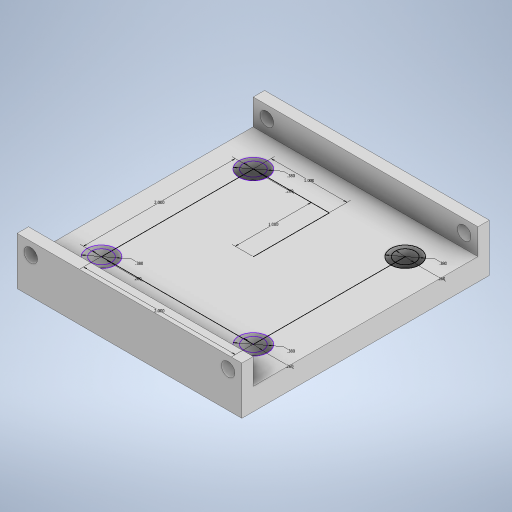
# Autodesk Inventor part: Voicecoil_to_PY004_Coupler
Saved by Autodesk Inventor 2024.2 (Build 282272000, 272)
## iProperties
Created: 2023-11-10
Part Number: Voicecoil_to_PY004_Coupler
Material: Generic
Document SubType Name: Modeling
Designer: S227943
Density: 1 g/cm^3
Appearance: Default
Author: S227943
Autodesk Inventor part; units mm, degrees
ref_plane "YZ Plane" through (0, 0, 0) normal (1, 0, 0) x (0, 1, 0)
ref_plane "XZ Plane" through (0, 0, 0) normal (0, 1, 0) x (-1, 0, 0)
ref_plane "XY Plane" through (0, 0, 0) normal (0, 0, 1) x (1, 0, 0)
sketch "Sketch1" plane through (0, 0, 0) normal (0, 1, 0) x (-1, 0, 0)
  line L0 (37.592, 37.592) -> (-37.592, 37.592)
  line L1 (-37.592, 37.592) -> (-37.592, -37.592)
  line L2 (-37.592, -37.592) -> (37.592, -37.592)
  line L3 (37.592, -37.592) -> (37.592, 37.592)
  line L4 (48.9249, 50.7063) -> (48.9249, -4.5387)
  line L5 (37.592, 0) -> (0, 0)
  line L6 (0, 0) -> (0, -37.592)
  point P0 (0, 0)
  dimension "d0" = 75.184
  dimension "d1" = 75.184
  constraints: 14 end point, 3 parallel, 2 midpoint, 1 horizontal, 1 perpendicular
  measures "d0" distance of L1.end L2.end
  measures "d1" distance of L0.end L1.end
extrude "Extrusion1" add sketch "Sketch1" along normal blind 7.366
sketch "Sketch6" plane through (0, 7.366, 0) normal (0, 1, 0) x (1, 0, 0)
  line L0 (0, 0) -> (0, 25.4)
  line L1 (0, 25.4) -> (-25.4, 25.4)
  line L2 (-25.4, 25.4) -> (-25.4, -25.4)
  line L3 (-25.4, -25.4) -> (25.4, -25.4)
  line L4 (25.4, -25.4) -> (25.4, 25.4)
  circle A0 centre (25.4, 25.4) radius 3.302
  circle A1 centre (25.4, 25.4) radius 4.826
  circle A2 centre (25.4, -25.4) radius 3.302
  circle A3 centre (25.4, -25.4) radius 4.826
  circle A4 centre (-25.4, -25.4) radius 3.302
  circle A5 centre (-25.4, -25.4) radius 4.826
  circle A6 centre (-25.4, 25.4) radius 3.302
  circle A7 centre (-25.4, 25.4) radius 4.826
  dimension "d35" = 25.4
  dimension "d36" = 25.4
  dimension "d37" = 50.8
  dimension "d38" = 50.8
  dimension "d39" = 6.604
  dimension "d40" = 9.652
  dimension "d41" = 6.604
  dimension "d42" = 9.652
  dimension "d43" = 6.604
  dimension "d44" = 9.652
  dimension "d45" = 6.604
  dimension "d46" = 9.652
  constraints: 10 end point, 8 centre point, 8 coincident, 4 perpendicular, 1 point on line, 1 vertical
  measures "d35" distance of L0.start L0.end
  measures "d36" distance of L0.end L1.end
  measures "d37" distance of L1.end L2.end
  measures "d38" distance of L2.end L3.end
  measures "d39" diameter of A0
  measures "d40" diameter of A1
  measures "d41" diameter of A2
  measures "d42" diameter of A3
  measures "d43" diameter of A4
  measures "d44" diameter of A5
  measures "d45" diameter of A6
  measures "d46" diameter of A7
sketch "Sketch2" plane through (0, 7.366, 0) normal (0, 1, 0) x (1, 0, 0)
  line L0 (0, 0) -> (0, 12.7)
  line L1 (0, 12.7) -> (-12.7, 12.7)
  line L2 (-12.7, 12.7) -> (12.7, 12.7)
  line L3 (12.7, 12.7) -> (12.7, -12.7)
  line L4 (12.7, -12.7) -> (-12.7, -12.7)
  circle A0 centre (-12.7, -12.7) radius 3.302
  circle A1 centre (-12.7, -12.7) radius 4.826
  circle A2 centre (-12.7, 12.7) radius 3.302
  circle A3 centre (-12.7, 12.7) radius 4.826
  circle A4 centre (12.7, -12.7) radius 3.302
  circle A5 centre (12.7, -12.7) radius 4.826
  circle A6 centre (12.7, 12.7) radius 3.302
  circle A7 centre (12.7, 12.7) radius 4.826
  dimension "d4" = 12.7
  dimension "d5" = 12.7
  dimension "d6" = 25.4
  dimension "d7" = 25.4
  dimension "d8" = 25.4
  dimension "d9" = 6.604
  dimension "d10" = 9.652
  dimension "d11" = 6.604
  dimension "d12" = 9.652
  dimension "d13" = 6.604
  dimension "d14" = 9.652
  dimension "d15" = 6.604
  dimension "d16" = 9.652
  constraints: 10 end point, 8 centre point, 5 coincident, 3 perpendicular, 1 point on line, 1 vertical
  measures "d4" distance of L0.start L0.end
  measures "d5" distance of L0.end L1.end
  measures "d6" distance of L1.end L2.end
  measures "d7" distance of L2.end L3.end
  measures "d8" distance of L3.end L4.end
  measures "d9" diameter of A0
  measures "d10" diameter of A1
  measures "d11" diameter of A2
  measures "d12" diameter of A3
  measures "d13" diameter of A4
  measures "d14" diameter of A5
  measures "d15" diameter of A6
  measures "d16" diameter of A7
sketch "Sketch3" plane through (-37.592, 0, 37.592) normal (0, 0, 1) x (1, 0, 0)
  point P0 (37.592, 0)
sketch "Sketch4" plane through (0, 0, 0) normal (0, -1, 0) x (1, 0, 0)
  line L0 (-37.592, 37.592) -> (38.608, 37.592)
  line L1 (38.608, 37.592) -> (38.608, 41.402)
  line L2 (38.608, 41.402) -> (-37.592, 41.402)
  line L3 (-37.592, 41.402) -> (-37.592, 37.592)
  line L4 (37.592, -37.592) -> (-37.592, -37.592) projected
  line L5 (-37.592, -37.592) -> (38.608, -37.592)
  line L6 (38.608, -37.592) -> (38.608, -41.402)
  line L7 (38.608, -41.402) -> (-37.592, -41.402)
  line L8 (-37.592, -41.402) -> (-37.592, -37.592)
  line L9 (37.592, 37.592) -> (37.592, 41.402)
  line L10 (37.592, -37.592) -> (37.592, -41.402)
  point P0 (0, 0)
  point P1 (38.1, -38.1)
  dimension "d21" = 3.81
  dimension "d22" = 3.81
  constraints: 20 end point, 5 point on line, 4 parallel, 3 perpendicular, 2 horizontal
  measures "d21" distance of L0.end L1.end
  measures "d22" distance of L5.end L6.end
extrude "Extrusion4" add sketch "Sketch4" against normal blind 16.002 contours L3 L2 L9 L0 | L10 L7 L8 L4
sketch "Sketch5" plane through (-37.592, 0, 41.402) normal (0, 0, 1) x (1, 0, 0)
  line L0 (0, 7.366) -> (75.184, 7.366) projected
  line L1 (75.184, 7.366) -> (70.612, 7.366)
  line L2 (70.612, 7.366) -> (70.612, 11.938)
  line L3 (0, 7.366) -> (4.572, 7.366)
  line L4 (4.572, 7.366) -> (4.572, 11.938)
  circle A0 centre (4.572, 11.938) radius 2.286
  circle A1 centre (70.612, 11.938) radius 2.286
  point P0 (37.592, 0)
  dimension "d25" = 4.572
  dimension "d26" = 4.572
  dimension "d27" = 4.572
  dimension "d51" = 4.572
  dimension "d52" = 4.572
  constraints: 8 end point, 2 centre point, 2 coincident, 2 perpendicular, 2 point on line
  measures "d25" distance of L0.end L1.end
  measures "d26" distance of L1.end L2.end
  measures "d27" distance of L0.start L3.end
  measures "d51" diameter of A0
  measures "d52" diameter of A1
extrude "Extrusion5" cut sketch "Sketch6" against normal blind 25.4 contours A0 | A6 L2 L1 | L1 L2 A6 | A4 L3 L2 | L2 L3 A4 | A2 L4 L3 | L3 L4 A2
extrude "Extrusion6" cut sketch "Sketch6" against normal blind 6.604 contours A7 L2 A6 L1 | L1 A6 L2 A7 | A0 | A1 | A3 L4 A2 L3 | L3 A2 L4 A3 | A5 L3 A4 L2 | L2 A4 L3 A5 | A6 L2 L1 | L1 L2 A6 | A4 L3 L2 | L2 L3 A4 | A2 L4 L3 | L3 L4 A2
extrude "Extrusion7" cut sketch "Sketch5" against normal blind 127
body "Solid1"
